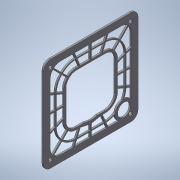
# Autodesk Inventor part: NewFront_F
Saved by Autodesk Inventor 2020 (Build 240168000, 168)
## iProperties
Created: 2019-07-06
Part Number: NewFront_F
Material: Generic
Document SubType Name: Modeling
Designer: DDeGo
Density: 1 g/cm^3
Appearance: Default
Author: DDeGo
Autodesk Inventor part; units mm, degrees
ref_plane "YZ Plane" through (0, 0, 0) normal (1, 0, 0) x (0, 1, 0)
ref_plane "XZ Plane" through (0, 0, 0) normal (0, 1, 0) x (-1, 0, 0)
ref_plane "XY Plane" through (0, 0, 0) normal (0, 0, 1) x (1, 0, 0)
sketch "Sketch1" plane through (0, 0, 0) normal (1, 0, 0) x (0, 1, 0)
  line L0 (0, 13.5) -> (156.2, 13.5)
  line L1 (169.7, 0) -> (169.7, -156.2)
  line L2 (156.2, -169.7) -> (0, -169.7)
  line L3 (-13.5, -156.2) -> (-13.5, 0)
  arc A0 (169.7, 0) -> (156.2, 13.5) centre (156.2, 0) ccw
  arc A1 (156.2, -169.7) -> (169.7, -156.2) centre (156.2, -156.2) ccw
  arc A2 (-13.5, -156.2) -> (0, -169.7) centre (0, -156.2) ccw
  arc A3 (0, 13.5) -> (-13.5, 0) centre (0, 0) ccw
  line L4 (19.5, 0.5) -> (136.7, 0.5)
  line L5 (156.7, -19.5) -> (156.7, -136.7)
  line L6 (136.7, -156.7) -> (19.5, -156.7)
  line L7 (-0.5, -136.7) -> (-0.5, -19.5)
  arc A4 (19.5, 0.5) -> (-0.5, -19.5) centre (19.5, -19.5) ccw
  arc A5 (-0.5, -136.7) -> (19.5, -156.7) centre (19.5, -136.7) ccw
  arc A6 (136.7, -156.7) -> (156.7, -136.7) centre (136.7, -136.7) ccw
  arc A7 (156.7, -19.5) -> (136.7, 0.5) centre (136.7, -19.5) ccw
  line L8 (156.2, 63.5) -> (0, 63.5)
  arc A8 (0, 63.5) -> (-63.5, 0) centre (0, 0) ccw
  line L9 (-63.5, 0) -> (-63.5, -156.2)
  arc A9 (-63.5, -156.2) -> (0, -219.7) centre (0, -156.2) ccw
  line L10 (0, -219.7) -> (156.2, -219.7)
  arc A10 (156.2, -219.7) -> (219.7, -156.2) centre (156.2, -156.2) ccw
  line L11 (219.7, -156.2) -> (219.7, 0)
  arc A11 (219.7, 0) -> (156.2, 63.5) centre (156.2, 0) ccw
  dimension "d0" = 13.5
  dimension "d1" = 183.2
  dimension "d2" = 183.2
  dimension "d15" = 13
  dimension "d16" = 13
  dimension "d17" = 13
  dimension "d18" = 13
  dimension "d19" = 20
  dimension "d41" = 50
  constraints: 24 end point, 24 point on circle, 16 tangent, 12 centre point, 6 equal radius, 6 parallel, 3 perpendicular, 2 horizontal, 8 other
  measures "d0" radius of A0
  measures "d1" distance between parallel lines of L2 L0
  measures "d2" distance between parallel lines of L1 L3
  measures "d15" distance between parallel lines of L3 L7
  measures "d16" distance between parallel lines of L0 L4
  measures "d17" distance between parallel lines of L1 L5
  measures "d18" distance between parallel lines of L2 L6
  measures "d19" radius of A4
  measures "d41" distance between parallel lines of L0 L8
extrude "Extrusion1" add sketch "Sketch1" along normal blind 3 contours L0 A0 L1 A1 L2 A2 L3 A3
sketch "Sketch3" plane through (3, 0, 0) normal (1, 0, 0) x (0, 0, -1)
  line L0 (106.1, 30.1) -> (50.1, 30.1)
  line L1 (30.1, 50.1) -> (30.1, 106.1)
  line L2 (50.1, 126.1) -> (106.1, 126.1)
  line L3 (126.1, 106.1) -> (126.1, 50.1)
  line L4 (126.1, 30.1) -> (30.1, 126.1) construction
  line L5 (30.1, 30.1) -> (126.1, 126.1) construction
  arc A0 (169.7, 156.2) -> (156.2, 169.7) centre (156.2, 156.2) ccw projected
  line L6 (0, 0) -> (156.2, 156.2) construction
  arc A1 (-0.5, 19.5) -> (19.5, -0.5) centre (19.5, 19.5) ccw projected
  line L7 (-0.5, 19.5) -> (-0.5, 136.7) projected
  arc A2 (19.5, 156.7) -> (-0.5, 136.7) centre (19.5, 136.7) ccw projected
  line L8 (19.5, 156.7) -> (136.7, 156.7) projected
  arc A3 (156.7, 136.7) -> (136.7, 156.7) centre (136.7, 136.7) ccw projected
  line L9 (156.7, 136.7) -> (156.7, 19.5) projected
  arc A4 (136.7, -0.5) -> (156.7, 19.5) centre (136.7, 19.5) ccw projected
  line L10 (136.7, -0.5) -> (19.5, -0.5) projected
  line L11 (156.2, 169.7) -> (0, 169.7) projected
  arc A5 (0, 169.7) -> (-13.5, 156.2) centre (0, 156.2) ccw projected
  line L12 (-13.5, 156.2) -> (-13.5, 0) projected
  arc A6 (-13.5, 0) -> (0, -13.5) centre (0, 0) ccw projected
  line L13 (0, -13.5) -> (156.2, -13.5) projected
  arc A7 (156.2, -13.5) -> (169.7, 0) centre (156.2, 0) ccw projected
  line L14 (169.7, 0) -> (169.7, 156.2) projected
  arc A8 (169.7, 156.2) -> (156.2, 169.7) centre (156.2, 156.2) ccw projected
  line L15 (30.1, 79.35) -> (-39.9, 79.35)
  line L16 (-39.9, 79.35) -> (-39.9, 76.85)
  line L17 (-39.9, 76.85) -> (30.1, 76.85)
  line L18 (30.1, 76.85) -> (30.1, 79.35)
  line L19 (30.1, 78.1) -> (78.1, 78.1) construction
  line L20 (34.2321, 58.5763) -> (33.2754, 60.886)
  line L21 (-30.4394, 31.7885) -> (34.2321, 58.5763)
  line L22 (33.2754, 60.886) -> (-31.3961, 34.0982)
  line L23 (-31.3961, 34.0982) -> (-30.4394, 31.7885)
  line L24 (45.0428, 43.275) -> (43.275, 45.0428)
  line L25 (-4.4547, -6.2225) -> (45.0428, 43.275)
  line L26 (43.275, 45.0428) -> (-6.2225, -4.4547)
  line L27 (-6.2225, -4.4547) -> (-4.4547, -6.2225)
  line L28 (60.886, 33.2754) -> (58.5763, 34.2321)
  line L29 (34.0982, -31.3961) -> (60.886, 33.2754)
  line L30 (58.5763, 34.2321) -> (31.7885, -30.4394)
  line L31 (31.7885, -30.4394) -> (34.0982, -31.3961)
  line L32 (79.35, 30.1) -> (76.85, 30.1)
  line L33 (79.35, -39.9) -> (79.35, 30.1)
  line L34 (76.85, 30.1) -> (76.85, -39.9)
  line L35 (76.85, -39.9) -> (79.35, -39.9)
  line L36 (97.6237, 34.2321) -> (95.314, 33.2754)
  line L37 (124.4115, -30.4394) -> (97.6237, 34.2321)
  line L38 (95.314, 33.2754) -> (122.1018, -31.3961)
  line L39 (122.1018, -31.3961) -> (124.4115, -30.4394)
  line L40 (112.925, 45.0428) -> (111.1572, 43.275)
  line L41 (162.4225, -4.4547) -> (112.925, 45.0428)
  line L42 (111.1572, 43.275) -> (160.6547, -6.2225)
  line L43 (160.6547, -6.2225) -> (162.4225, -4.4547)
  line L44 (122.9246, 60.886) -> (121.9679, 58.5763)
  line L45 (187.5961, 34.0982) -> (122.9246, 60.886)
  line L46 (121.9679, 58.5763) -> (186.6394, 31.7885)
  line L47 (186.6394, 31.7885) -> (187.5961, 34.0982)
  line L48 (126.1, 79.35) -> (126.1, 76.85)
  line L49 (196.1, 79.35) -> (126.1, 79.35)
  line L50 (126.1, 76.85) -> (196.1, 76.85)
  line L51 (196.1, 76.85) -> (196.1, 79.35)
  line L52 (121.9679, 97.6237) -> (122.9246, 95.314)
  line L53 (186.6394, 124.4115) -> (121.9679, 97.6237)
  line L54 (122.9246, 95.314) -> (187.5961, 122.1018)
  line L55 (187.5961, 122.1018) -> (186.6394, 124.4115)
  line L56 (111.1572, 112.925) -> (112.925, 111.1572)
  line L57 (160.6547, 162.4225) -> (111.1572, 112.925)
  line L58 (112.925, 111.1572) -> (162.4225, 160.6547)
  line L59 (162.4225, 160.6547) -> (160.6547, 162.4225)
  line L60 (95.314, 122.9246) -> (97.6237, 121.9679)
  line L61 (122.1018, 187.5961) -> (95.314, 122.9246)
  line L62 (97.6237, 121.9679) -> (124.4115, 186.6394)
  line L63 (124.4115, 186.6394) -> (122.1018, 187.5961)
  line L64 (76.85, 126.1) -> (79.35, 126.1)
  line L65 (76.85, 196.1) -> (76.85, 126.1)
  line L66 (79.35, 126.1) -> (79.35, 196.1)
  line L67 (79.35, 196.1) -> (76.85, 196.1)
  line L68 (58.5763, 121.9679) -> (60.886, 122.9246)
  line L69 (31.7885, 186.6394) -> (58.5763, 121.9679)
  line L70 (60.886, 122.9246) -> (34.0982, 187.5961)
  line L71 (34.0982, 187.5961) -> (31.7885, 186.6394)
  line L72 (43.275, 111.1572) -> (45.0428, 112.925)
  line L73 (-6.2225, 160.6547) -> (43.275, 111.1572)
  line L74 (45.0428, 112.925) -> (-4.4547, 162.4225)
  line L75 (-4.4547, 162.4225) -> (-6.2225, 160.6547)
  line L76 (33.2754, 95.314) -> (34.2321, 97.6237)
  line L77 (-31.3961, 122.1018) -> (33.2754, 95.314)
  line L78 (34.2321, 97.6237) -> (-30.4394, 124.4115)
  line L79 (-30.4394, 124.4115) -> (-31.3961, 122.1018)
  arc A9 (50.1, 126.1) -> (30.1, 106.1) centre (50.1, 106.1) ccw
  arc A10 (30.1, 50.1) -> (50.1, 30.1) centre (50.1, 50.1) ccw
  arc A11 (106.1, 30.1) -> (126.1, 50.1) centre (106.1, 50.1) ccw
  arc A12 (126.1, 106.1) -> (106.1, 126.1) centre (106.1, 106.1) ccw
  line L80 (9.5, 106.1) -> (9.5, 50.1)
  arc A13 (9.5, 50.1) -> (50.1, 9.5) centre (50.1, 50.1) ccw
  line L81 (50.1, 9.5) -> (106.1, 9.5)
  arc A14 (106.1, 9.5) -> (146.7, 50.1) centre (106.1, 50.1) ccw
  line L82 (146.7, 50.1) -> (146.7, 106.1)
  arc A15 (146.7, 106.1) -> (106.1, 146.7) centre (106.1, 106.1) ccw
  line L83 (106.1, 146.7) -> (50.1, 146.7)
  arc A16 (50.1, 146.7) -> (9.5, 106.1) centre (50.1, 106.1) ccw
  line L84 (11.5, 106.1) -> (11.5, 50.1)
  arc A17 (11.5, 50.1) -> (50.1, 11.5) centre (50.1, 50.1) ccw
  line L85 (50.1, 11.5) -> (106.1, 11.5)
  arc A18 (106.1, 11.5) -> (144.7, 50.1) centre (106.1, 50.1) ccw
  line L86 (144.7, 50.1) -> (144.7, 106.1)
  arc A19 (144.7, 106.1) -> (106.1, 144.7) centre (106.1, 106.1) ccw
  line L87 (106.1, 144.7) -> (50.1, 144.7)
  arc A20 (50.1, 144.7) -> (11.5, 106.1) centre (50.1, 106.1) ccw
  line L88 (83.1, 68.1) -> (73.1, 68.1)
  line L89 (73.1, 68.1) -> (73.1, 88.1)
  line L90 (73.1, 88.1) -> (83.1, 88.1)
  line L91 (83.1, 88.1) -> (83.1, 68.1)
  line L92 (83.1, 68.1) -> (73.1, 88.1) construction
  line L93 (73.1, 68.1) -> (83.1, 88.1) construction
  line L94 (26.1, 106.1) -> (26.1, 50.1)
  arc A21 (26.1, 50.1) -> (50.1, 26.1) centre (50.1, 50.1) ccw
  line L95 (50.1, 26.1) -> (106.1, 26.1)
  arc A22 (106.1, 26.1) -> (130.1, 50.1) centre (106.1, 50.1) ccw
  line L96 (130.1, 50.1) -> (130.1, 106.1)
  arc A23 (130.1, 106.1) -> (106.1, 130.1) centre (106.1, 106.1) ccw
  line L97 (106.1, 130.1) -> (50.1, 130.1)
  arc A24 (50.1, 130.1) -> (26.1, 106.1) centre (50.1, 106.1) ccw
  point P0 (33.7538, 59.7312)
  point P1 (44.1589, 44.1589)
  point P2 (59.7312, 33.7538)
  point P3 (78.1, 30.1)
  point P4 (96.4688, 33.7538)
  point P5 (112.0411, 44.1589)
  point P6 (122.4462, 59.7312)
  point P7 (126.1, 78.1)
  point P8 (122.4462, 96.4688)
  point P9 (112.0411, 112.0411)
  point P10 (96.4688, 122.4462)
  point P11 (78.1, 126.1)
  point P12 (59.7312, 122.4462)
  point P13 (44.1589, 112.0411)
  point P14 (33.7538, 96.4688)
  dimension "d28" = 96
  dimension "d29" = 96
  dimension "d30" = 2.5
  dimension "d31" = 70
  dimension "d34" = 360
  dimension "d38" = 20
  dimension "d39" = 2
  dimension "d40" = 10
  dimension "d44" = 10
  dimension "d45" = 20
  dimension "d61" = 4
  constraints: 180 end point, 32 point on circle, 16 centre point, 12 parallel, 9 point on line, 8 tangent, 6 midpoint, 6 perpendicular, 4 horizontal, 3 equal radius, 166 other
  measures "d28" distance of L4.end L5.end
  measures "d29" distance of L5.end L4.start
  measures "d30" distance of L15.end L16.end
  measures "d31" distance of L15.start L15.end
  measures "d38" radius of A9
  measures "d39" distance between parallel lines of L80 L84
  measures "d40" distance between parallel lines of L7 L80
  measures "d44" distance of L89.end L90.end
  measures "d45" distance of L88.end L89.end
  measures "d61" distance between parallel lines of L1 L94
extrude "Extrusion3" add sketch "Sketch3" against normal up to surface (3 mm away) contours L33 L95 L34 L0 | L0 L38 L95 L33 | L34 L95 L29 L0 | L38 L36 L37 L0 | L0 L37 L95 L38 | L33 L85 L34 L95 | L29 L95 L30 L0 | L0 L30 L28 L29 | L0 A11 L42 A22 L95 L37 | L95 L37 A18 L85 L38 | L85 L38 L81 L33 | L33 L81 L34 L85 | L30 L95 A21 L25 A10 L0 | L29 L85 A17 L30 L95 | L34 L81 L29 L85 | L85 A18 L37 A14 L81 L38 | L33 L10 L34 L81 | L29 L81 A13 L30 A17 L85 | A11 L41 A22 L42 | L42 L40 L41 A11 | A18 L42 A14 L37 | L81 A14 L37 L10 L38 | L33 L13 L34 L10 | A10 L26 L24 L25 | L25 A21 L26 A10 | L30 A13 L25 A17 | L29 L10 L30 A13 L81 | A22 L41 A18 L42 | A11 L3 L46 L96 A22 L41 | A18 L41 A14 L42 | L10 L37 L13 L38 | L33 L35 L34 L13 | L25 A17 L26 A21 | L26 A21 L94 L21 L1 A10 | L25 A13 L26 A17 | L29 L13 L30 L10 | A14 L41 A4 L42 | A18 L46 A14 L41 | L13 L37 L39 L38 | L25 A1 L26 A13 | L26 A13 L21 A17 | L29 L31 L30 L13 | L46 L44 L45 L3 | L3 L45 L96 L46 | A4 L41 L43 L42 | A18 L86 L45 L82 A14 L46 | L46 L96 L45 L86 A18 | L21 L94 L22 L1 | L1 L22 L20 L21 | L25 L27 L26 A1 | A17 L84 L22 L94 L21 | L21 A13 L80 L22 L84 A17 | L3 L50 L96 L45 | A14 L82 L45 L9 L46 | L22 L94 L17 L1 | L21 L7 L22 L80 A13 | L3 L49 L96 L50 | L9 L45 L14 L46 | L86 L50 L82 L45 | L17 L94 L15 L1 | L21 L12 L22 L7 | L22 L80 L17 L84 | L96 L49 L86 L50 | L3 L54 L96 L49 | L14 L45 L47 L46 | L86 L49 L82 L50 | L17 L84 L15 L94 | L15 L94 L77 L1 | L21 L23 L22 L12 | L17 L80 L15 L84 | L54 L52 L53 L3 | L3 L53 L96 L54 | L50 L82 L49 L9 | L9 L49 L14 L50 | L86 L54 L82 L49 | L77 L94 L78 L1 | L1 L78 L76 L77 | L17 L12 L15 L7 | L7 L15 L80 L17 | L15 L80 L77 L84 | L96 L53 A19 L86 L54 | L3 A12 L58 A23 L96 L53 | L14 L49 L51 L50 | L86 A19 L53 A15 L82 L54 | L77 L84 A20 L78 L94 | L78 L94 A24 L73 A9 L1 | L17 L16 L15 L12 | L77 L80 A16 L78 A20 L84 | L54 L82 A15 L53 L9 | L9 L53 L14 L54 | L77 L12 L78 L7 | L7 L78 A16 L80 L77 | A19 L58 A15 L53 | A12 L57 A23 L58 | L14 L53 L55 L54 | L78 A16 L73 A20 | A9 L74 L72 L73 | L73 A24 L74 A9 | L77 L79 L78 L12 | A19 L57 A15 L58 | A12 L2 L62 L97 A23 L57 | A20 L74 A24 L73 | L73 A16 L74 A20 | L74 A24 L97 L69 L2 A9 | A19 L62 A15 L57 | L73 A2 L74 A16 | L74 A16 L69 A20 | L73 L75 L74 A2 | A19 L87 L61 L83 A15 L62 | L62 L97 L61 L87 A19 | L62 L60 L61 L2 | L2 L61 L97 L62 | A20 L87 L70 L97 L69 | L69 A16 L83 L70 L87 A20 | L69 L97 L70 L2 | L2 L70 L68 L69 | A15 L83 L61 L8 L62 | L2 L66 L97 L61 | L62 L8 L61 L11 | L11 L61 L63 L62 | L69 L8 L70 L83 A16 | L70 L97 L65 L2 | L69 L71 L70 L11 | L11 L70 L8 L69 | L87 L66 L83 L61 | L2 L65 L97 L66 | L70 L83 L65 L87 | L97 L65 L87 L66 | L87 L65 L83 L66 | L66 L8 L65 L11 | L11 L65 L67 L66 | L66 L83 L65 L8
extrude "Extrusion4" cut sketch "Sketch1" along normal blind 10 contours A11 L11 A10 L10 A9 L9 A8 L8
sketch "Sketch4" plane through (0, 0, 0) normal (-1, 0, 0) x (0, 0, 1)
  circle A0 centre (-142.7, 142.7) radius 12.5
  circle A1 centre (-142.7, 142.7) radius 17.5
  line L0 (-156.2, 169.7) -> (0, 169.7) projected
  line L1 (-169.7, 0) -> (-169.7, 156.2) projected
  line L2 (-112.0102, 156.7) -> (-136.7, 156.7) projected
  arc A2 (-107.0349, 144.6887) -> (-144.6887, 107.0349) centre (-106.1, 106.1) ccw projected
  line L3 (-79.5219, 78.1077) -> (-78.1077, 79.5219)
  line L4 (-78.1077, 79.5219) -> (-91.2684, 92.6827)
  line L5 (-91.2684, 92.6827) -> (-92.6827, 91.2684)
  line L6 (-92.6827, 91.2684) -> (-79.5219, 78.1077)
  arc A3 (-106.1, 126.1) -> (-126.1, 106.1) centre (-106.1, 106.1) ccw projected
  arc A4 (-106.1, 126.1) -> (-126.1, 106.1) centre (-106.1, 106.1) ccw projected
  line L7 (-91.9756, 91.9756) -> (-106.1, 106.1) construction
  line L8 (-126.1, 50.1) -> (-126.1, 56.8648) projected
  point P0 (0, 0)
  point P1 (-105.5, 141)
  point P2 (-141, 105.5)
  point P3 (-105.5, 125.5)
  point P4 (-125.5, 105.5)
  point P5 (-125.5, 99.0281)
  dimension "d46" = 27
  dimension "d47" = 27
  dimension "d48" = 5
  dimension "d52" = 45
  dimension "d53" = 2
  dimension "d67" = 25
  constraints: 10 end point, 2 centre point, 2 parallel, 1 coincident, 1 midpoint, 1 perpendicular, 7 other
  measures "d46" distance from line of L0 A0.centre
  measures "d47" distance from line of L1 A0.centre
  measures "d48" radial gap between concentric circles of A1 A0
  measures "d52" angle to the sketch x axis of L7
  measures "d53" distance between parallel lines of L6 L4
  measures "d67" diameter of A0
extrude "Extrusion5" add sketch "Sketch4" against normal up to surface (3 mm away)
fillet "Fillet1" radius 1.5 2 edges at (1.5, 141.9173, -125.2175) (1.5, 125.2175, -141.9173)
sketch "Sketch5" plane through (0, 0, 0) normal (-1, 0, 0) x (0, 0, 1)
  line L0 (-0.5, 0.5) -> (-155.7, 0.5) construction
  line L1 (-155.7, 0.5) -> (-155.7, 155.7) construction
  line L2 (-155.7, 155.7) -> (-0.5, 155.7) construction
  line L3 (-0.5, 155.7) -> (-0.5, 0.5) construction
  line L4 (-3.625, 158.825) -> (2.625, 158.825)
  line L5 (2.625, 158.825) -> (2.625, 152.575)
  line L6 (2.625, 152.575) -> (-3.625, 152.575)
  line L7 (-3.625, 152.575) -> (-3.625, 158.825)
  line L8 (-3.625, 158.825) -> (2.625, 152.575) construction
  line L9 (2.625, 158.825) -> (-3.625, 152.575) construction
  line L10 (-3.625, 3.625) -> (2.625, 3.625)
  line L11 (2.625, 3.625) -> (2.625, -2.625)
  line L12 (2.625, -2.625) -> (-3.625, -2.625)
  line L13 (-3.625, -2.625) -> (-3.625, 3.625)
  line L14 (-3.625, 3.625) -> (2.625, -2.625) construction
  line L15 (2.625, 3.625) -> (-3.625, -2.625) construction
  line L16 (-158.825, 3.625) -> (-152.575, 3.625)
  line L17 (-152.575, 3.625) -> (-152.575, -2.625)
  line L18 (-152.575, -2.625) -> (-158.825, -2.625)
  line L19 (-158.825, -2.625) -> (-158.825, 3.625)
  line L20 (-158.825, 3.625) -> (-152.575, -2.625) construction
  line L21 (-152.575, 3.625) -> (-158.825, -2.625) construction
  line L22 (-152.575, 152.575) -> (-158.825, 152.575)
  line L23 (-158.825, 152.575) -> (-158.825, 158.825)
  line L24 (-158.825, 158.825) -> (-152.575, 158.825)
  line L25 (-152.575, 158.825) -> (-152.575, 152.575)
  line L26 (-152.575, 152.575) -> (-158.825, 158.825) construction
  line L27 (-158.825, 152.575) -> (-152.575, 158.825) construction
  line L28 (-156.2, -13.5) -> (0, -13.5) projected
  line L29 (-169.7, 156.2) -> (-169.7, 0) projected
  line L30 (13.5, 0) -> (13.5, 156.2) projected
  line L31 (0, 169.7) -> (-156.2, 169.7) projected
  point P0 (0, 0)
  dimension "d54" = 6.25
  dimension "d55" = 14
  dimension "d56" = 14
  dimension "d57" = 14
  dimension "d58" = 14
  constraints: 56 end point, 10 parallel, 8 midpoint, 7 equal length, 5 horizontal, 5 perpendicular
  measures "d54" distance of L4.start L4.end
  measures "d55" distance between parallel lines of L28 L0
  measures "d56" distance between parallel lines of L29 L1
  measures "d57" distance between parallel lines of L30 L3
  measures "d58" distance between parallel lines of L31 L2
extrude "Extrusion6" cut sketch "Sketch5" against normal blind 10
sketch "Sketch6" plane through (3, 0, 0) normal (1, 0, 0) x (0, 0, -1)
  line L0 (50.1, 30.1) -> (106.1, 30.1)
  line L1 (126.1, 50.1) -> (126.1, 106.1)
  line L2 (106.1, 126.1) -> (50.1, 126.1)
  line L3 (30.1, 106.1) -> (30.1, 50.1)
  line L4 (30.1, 59.5707) -> (30.1, 96.6293) projected
  line L5 (59.5707, 126.1) -> (96.6293, 126.1) projected
  line L6 (126.1, 96.6293) -> (126.1, 59.5707) projected
  line L7 (96.6293, 30.1) -> (59.5707, 30.1) projected
  arc A0 (30.1, 50.1) -> (50.1, 30.1) centre (50.1, 50.1) ccw
  arc A1 (50.1, 126.1) -> (30.1, 106.1) centre (50.1, 106.1) ccw
  arc A2 (126.1, 106.1) -> (106.1, 126.1) centre (106.1, 106.1) ccw
  arc A3 (106.1, 30.1) -> (126.1, 50.1) centre (106.1, 50.1) ccw
  point P0 (0, 0)
  dimension "d62" = 20
  constraints: 8 end point, 8 point on circle, 8 tangent, 4 centre point, 4 collinear, 3 equal radius, 2 parallel, 1 horizontal, 1 perpendicular
  measures "d62" radius of A0
extrude "Extrusion7" cut sketch "Sketch6" against normal blind 10
sketch "Sketch7" plane through (3, 0, 0) normal (1, 0, 0) x (0, 0, -1)
  arc A0 (144.6685, 155.044) -> (131.0727, 138.1113) centre (142.7, 142.7) ccw projected
  circle A1 centre (142.7, 142.7) radius 12.5
  point P0 (0, 0)
  point P1 (152.375, 152.4239)
  constraints: 1 coincident, 4 other
extrude "Extrusion8" cut sketch "Sketch7" against normal blind 10
sketch "Sketch8" plane through (3, 0, 0) normal (1, 0, 0) x (0, 0, -1)
  line L0 (130.1, 76.85) -> (130.1, 57.9139) projected
  line L1 (130.1, 57.9139) -> (134.1, 76.85)
  line L2 (144.7, 76.85) -> (130.1, 76.85) projected
  line L3 (134.1, 76.85) -> (134.1, 79.35)
  line L4 (130.1, 79.35) -> (144.7, 79.35) projected
  line L5 (144.7, 104.3336) -> (130.1, 98.2861) projected
  line L6 (134.1, 79.35) -> (130.1, 98.2861)
  line L7 (130.1, 76.85) -> (130.1, 57.9139) projected
  line L8 (130.1, 98.2861) -> (130.1, 57.9139)
  point P0 (0, 0)
  dimension "d68" = 4
  constraints: 8 end point, 2 point on line, 1 collinear, 1 vertical
  measures "d68" distance between parallel lines of L8 L3
extrude "Extrusion9" add sketch "Sketch8" against normal up to surface (3 mm away)
sketch "Sketch9" plane through (3, 0, 0) normal (1, 0, 0) x (0, 0, -1)
  line L0 (126.1, 50.1) -> (126.1, 106.1) projected
  line L1 (126.1, 65.6) -> (128.2124, 75.6)
  line L2 (128.2124, 75.6) -> (128.2124, 80.6)
  line L3 (128.2124, 80.6) -> (126.1, 90.6)
  line L4 (126.1, 65.6) -> (126.1, 90.6)
  line L5 (134.1, 79.35) -> (130.1, 98.2861) projected
  line L6 (130.1, 57.9139) -> (134.1, 76.85) projected
  line L7 (144.7, 76.85) -> (134.1, 76.85) projected
  line L8 (134.1, 79.35) -> (144.7, 79.35) projected
  line L9 (134.1, 76.85) -> (134.1, 79.35)
  line L10 (134.1, 78.1) -> (128.2124, 78.1) construction
  point P0 (0, 0)
  dimension "d71" = 25
  dimension "d72" = 5
  constraints: 12 end point, 4 parallel, 2 midpoint, 2 point on line, 1 horizontal, 1 vertical
  measures "d71" distance of L3.end L1.start
  measures "d72" distance of L1.end L2.end
extrude "Extrusion10" cut sketch "Sketch9" against normal blind 10
equation "\"d1\" = d2"
equation "\"d16\" = d15"
equation "\"d17\" = d15"
equation "\"d18\" = d15"
equation "\"d29\" = d28"
equation "\"d56\" = d55"
equation "\"d57\" = d55"
equation "\"d58\" = d55"
body "Solid1"
